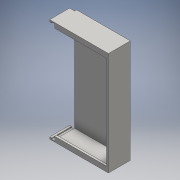
# Autodesk Inventor part: LEDs_protect
Saved by Autodesk Inventor 2016 (Build 200138000, 138)
## iProperties
Created: 2015-10-21
Part Number: LEDs_protect
Material: Generic
Document SubType Name: Modeling
Designer: fei
Density: 1 g/cm^3
Appearance: Default
Author: fei
Autodesk Inventor part; units mm, degrees
ref_plane "YZ Plane" through (0, 0, 0) normal (1, 0, 0) x (0, 1, 0)
ref_plane "XZ Plane" through (0, 0, 0) normal (0, 1, 0) x (-1, 0, 0)
ref_plane "XY Plane" through (0, 0, 0) normal (0, 0, 1) x (1, 0, 0)
sketch "Sketch1" plane through (0, 0, 0) normal (1, 0, 0) x (0, 1, 0)
  line L0 (10, 52) -> (-10, 52)
  line L1 (-10, 52) -> (-10, -52)
  line L2 (-10, -52) -> (10, -52)
  line L3 (10, -52) -> (10, 52)
  point P0 (0, 0)
  dimension "d0" = 104
  dimension "d1" = 20
  dimension "d2" = 52
  dimension "d3" = 10
  constraints: 8 end point, 2 parallel, 1 horizontal, 1 perpendicular
  measures "d0" distance of L2.end L0.start
  measures "d1" distance of L1.end L2.end
  measures "d2" distance from line of L2 point (0, 0)
  measures "d3" distance from line of L3 point (0, 0)
extrude "Extrusion1" add sketch "Sketch1" against normal blind 2
sketch "Sketch2" plane through (-2, 0, 0) normal (-1, 0, 0) x (0, 0, 1)
  line L0 (52, 10) -> (-52, 10) projected
  line L1 (-52, -10) -> (52, -10) projected
  line L2 (-52, 10) -> (-50, 10)
  line L3 (-50, 10) -> (-50, -10)
  line L4 (-50, -10) -> (-52, -10)
  line L5 (-52, -10) -> (-52, 10)
  line L6 (52, -10) -> (52, 10) projected
  line L7 (52, 10) -> (50, 10)
  line L8 (50, 10) -> (50, -10)
  line L9 (50, -10) -> (52, -10)
  line L10 (52, -10) -> (52, 10)
  point P0 (0, 0)
  dimension "d6" = 2
  dimension "d7" = 2
  constraints: 16 end point, 4 parallel, 2 horizontal, 2 perpendicular, 2 point on line
  measures "d6" distance between parallel lines of L5 L3
  measures "d7" distance between parallel lines of L6 L8
extrude "Extrusion2" add sketch "Sketch2" along normal blind 57 contours L6 L1 L8 L0 | L3 L1 L5 L0
sketch "Sketch3" plane through (0, 0, 0) normal (1, 0, 0) x (0, 0, -1)
  line L0 (52, 10) -> (-52, 10) projected
  line L1 (52, 10) -> (-52, 10)
  line L2 (-52, 10) -> (-52, 12)
  line L3 (-52, 12) -> (52, 12)
  line L4 (52, 12) -> (52, 10)
  line L5 (-52, 10) -> (-52, -10) projected
  point P0 (0, 0)
  dimension "d10" = 2
  dimension "d11" = 0
  constraints: 8 end point, 2 parallel, 1 horizontal, 1 perpendicular
  measures "d10" distance between parallel lines of L3 L0
  measures "d11" distance between parallel lines of L5 L2
extrude "Extrusion3" add sketch "Sketch3" against normal blind 54
sketch "Sketch6" plane through (-2, -10, 50) normal (0, 0, -1) x (-1, 0, 0)
  line L0 (52, 20) -> (57, 20) projected
  line L1 (0, 0) -> (57, 0) projected
  line L2 (52, 20) -> (55, 20)
  line L3 (55, 20) -> (55, 0)
  line L4 (55, 0) -> (52, 0)
  line L5 (52, 0) -> (52, 20)
  line L6 (57, 20) -> (57, 0) projected
  point P0 (-2, 10)
  dimension "d16" = 2
  dimension "d17" = 3
  constraints: 8 end point, 2 parallel, 2 point on line, 1 horizontal, 1 perpendicular
  measures "d16" distance between parallel lines of L6 L3
  measures "d17" distance between parallel lines of L5 L3
sketch "Sketch7" plane through (-59, -10, -50) normal (0, 0, 1) x (1, 0, 0)
  line L0 (5, 20) -> (0, 20) projected
  line L1 (59, 0) -> (0, 0) projected
  line L2 (2, 20) -> (5, 20)
  line L3 (5, 20) -> (5, 0)
  line L4 (5, 0) -> (2, 0)
  line L5 (2, 0) -> (2, 20)
  line L6 (0, 0) -> (0, 20) projected
  point P0 (59, 10)
  dimension "d18" = 3
  dimension "d19" = 2
  constraints: 8 end point, 2 parallel, 2 point on line, 1 horizontal, 1 perpendicular
  measures "d18" distance between parallel lines of L5 L3
  measures "d19" distance between parallel lines of L6 L5
extrude "Extrusion4" cut sketch "Sketch7" against normal blind 1 contours L3 L1 L5 L0
extrude "Extrusion5" cut sketch "Sketch6" against normal blind 1 contours L0 L3 L1 L5
sketch "Sketch8" plane through (-2, -10, -50) normal (0, 0, 1) x (1, 0, 0)
  line L0 (-52, 20) -> (-52, 0) projected
  line L1 (0, 0) -> (-52, 0)
  line L2 (-52, 0) -> (-52, 2)
  line L3 (-52, 2) -> (0, 2)
  line L4 (0, 2) -> (0, 0)
  point P0 (2, 10)
  dimension "d24" = 2
  constraints: 8 end point, 2 parallel, 1 coincident, 1 horizontal, 1 perpendicular, 1 point on line
  measures "d24" distance between parallel lines of L1 L3
sketch "Sketch9" plane through (-2, -10, 50) normal (0, 0, -1) x (-1, 0, 0)
  line L0 (52, 0) -> (0, 0)
  line L1 (0, 0) -> (0, 2)
  line L2 (0, 2) -> (52, 2)
  line L3 (52, 2) -> (52, 0)
  point P0 (-2, 10)
  dimension "d25" = 2
  constraints: 8 end point, 2 parallel, 1 coincident, 1 horizontal, 1 perpendicular
  measures "d25" distance between parallel lines of L0 L2
extrude "Extrusion6" add sketch "Sketch8" along normal blind 3
extrude "Extrusion7" add sketch "Sketch9" along normal blind 3
body "Solid1"
